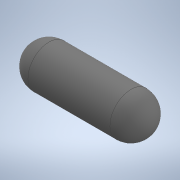
# Autodesk Inventor part: Cylinder
Saved by Autodesk Inventor 2020 (Build 240168000, 168)
## iProperties
Created: 2021-08-07
Part Number: Cylinder
Material: Fiberglass Batt
Document SubType Name: Modeling
Designer: Bisqwit2.0
Density: 0.032 g/cm^3
Appearance: Gray
Author: Bisqwit2.0
Autodesk Inventor part; units mm, degrees
ref_plane "YZ Plane" through (0, 0, 0) normal (1, 0, 0) x (0, 1, 0)
ref_plane "XZ Plane" through (0, 0, 0) normal (0, 1, 0) x (-1, 0, 0)
ref_plane "XY Plane" through (0, 0, 0) normal (0, 0, 1) x (1, 0, 0)
sketch "Sketch1" plane through (0, 0, 0) normal (0, 0, 1) x (1, 0, 0)
  line L0 (-1500, 0) -> (1500, 0)
  arc A0 (-1100, 400) -> (-1500, 0) centre (-1100, 0) ccw
  arc A1 (1500, 0) -> (1100, 400) centre (1100, 0) ccw
  line L1 (-1100, 400) -> (1100, 400)
  arc A2 (-1100, 565.078) -> (-1665.078, 0) centre (-1100, 0) ccw
  arc A3 (1665.078, 0) -> (1100, 565.078) centre (1100, 0) ccw
  line L2 (-1665.078, 0) -> (-1500, 0)
  line L3 (-1100, 565.078) -> (1100, 565.078)
  line L4 (1500, 0) -> (1665.078, 0)
  point P0 (0, 0)
  dimension "d0" = 3000
  dimension "d1" = 800
  dimension "d2" = 800
  dimension "d3" = 1100
  dimension "d4" = 1100
  dimension "d5" = 1130.156
  dimension "d6" = 1130.156
  constraints: 10 end point, 9 point on circle, 5 horizontal, 4 centre point, 3 point on line, 2 coincident, 2 tangent
  measures "d0" distance of L0.end L0.start
  measures "d1" diameter of A0
  measures "d2" diameter of A1
  measures "d3" distance of point (0, 0) A0.centre
  measures "d4" distance of point (0, 0) A1.centre
  measures "d5" diameter of A2
  measures "d6" diameter of A3
revolve "Revolution2" add sketch "Sketch1" angle 360 about axis through (-1500, 0, 0) along (1, 0, 0) contours L2 A2 L3 A3 L4 A1 L1 A0
body "Solid2"
